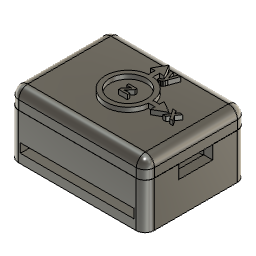
Tremolomter accel case (Autodesk Fusion 360 design; units mm, degrees)
Autodesk Fusion 360 part; units mm, degrees
sketch "Sketch1" plane through (0, 0, 0) normal (0, 0, 1) x (1, 0, 0)
  line L0 (0, 0) -> (29.9, 0)
  line L1 (29.9, 0) -> (29.9, 22.28)
  line L2 (29.9, 22.28) -> (0, 22.28)
  line L3 (0, 22.28) -> (0, 0)
  dimension "d4" = 29.9
  dimension "d5" = 22.28
  constraint horizontal L0
  constraint vertical L1
  constraint horizontal L2
  constraint vertical L3
  constraint coincident L0.start L3.end
  measures "d4" distance of L0.start L0.end
  measures "d5" distance of L0.start L2.end
extrude "Extrude1" add sketch "Sketch1" along normal blind 2 makes body 1
sketch "Sketch2" plane through (0, 0, 2) normal (0, 0, 1) x (-1, 0, 0)
  line L0 (0, -22.28) -> (0, 0)
  line L1 (0, 0) -> (-29.9, 0)
  line L2 (-29.9, 0) -> (-29.9, -22.28)
  line L3 (-29.9, -22.28) -> (0, -22.28)
  line L4 (-2, -2) -> (-27.9, -2)
  line L5 (-27.9, -2) -> (-27.9, -20.28)
  line L6 (-27.9, -20.28) -> (-2, -20.28)
  line L7 (-2, -20.28) -> (-2, -2)
  dimension "d9" = 25.9
  dimension "d10" = 18.28
  dimension "d11" = 2
  dimension "d12" = 2
  constraint horizontal L4
  constraint vertical L5
  constraint horizontal L6
  constraint vertical L7
  measures "d9" distance of L4.start L4.end
  measures "d10" distance of L4.start L6.end
  measures "d11" distance of L0 L7
  measures "d12" distance of L1 L4
extrude "Extrude2" add sketch "Sketch2" along normal blind 5 bodies 1
sketch "Sketch3" plane through (29.9, 0, 0) normal (1, 0, 0) x (0, 1, 0)
  line L0 (0, 0) -> (22.28, 0)
  line L1 (22.28, 0) -> (22.28, 7)
  line L2 (22.28, 7) -> (0, 7)
  line L3 (0, 7) -> (0, 0)
  line L4 (7.39, 4) -> (14.89, 4)
  line L5 (14.89, 4) -> (14.89, 7)
  line L6 (14.89, 7) -> (7.39, 7)
  line L7 (7.39, 7) -> (7.39, 4)
  dimension "d17" = 7.5
  dimension "d18" = 3
  dimension "d19" = 4
  dimension "d20" = 7.39
  constraint horizontal L4
  constraint vertical L5
  constraint horizontal L6
  constraint vertical L7
  measures "d17" distance of L4.start L4.end
  measures "d18" distance of L4.start L6.end
  measures "d19" distance of L0 L4
  measures "d20" distance of L3 L7
extrude "Extrude3" cut sketch "Sketch3" against normal blind 14 contours L2 L4 L5 L6 L7 bodies 1
sketch "Sketch4" plane through (0, 0, 2) normal (0, 0, 1) x (-1, 0, 0)
  line L0 (-2, -2) -> (-27.9, -2)
  line L1 (-27.9, -2) -> (-27.9, -20.28)
  line L2 (-27.9, -20.28) -> (-2, -20.28)
  line L3 (-2, -20.28) -> (-2, -2)
  circle A0 centre (-4.54, -17.74) radius 1
  circle A1 centre (-25.36, -17.74) radius 1
  circle A2 centre (-4.54, -4.54) radius 1
  circle A3 centre (-25.36, -4.54) radius 1
  dimension "d26" = 2
  dimension "d27" = 2.54
  dimension "d28" = 2.54
  dimension "d29" = 2
  dimension "d30" = 2.54
  dimension "d31" = 2.54
  dimension "d32" = 2
  dimension "d33" = 2.54
  dimension "d34" = 2.54
  dimension "d35" = 2
  dimension "d36" = 2.54
  dimension "d37" = 2.54
  measures "d26" diameter of A0
  measures "d27" distance of L2 A0.centre
  measures "d28" distance of L3 A0.centre
  measures "d29" diameter of A1
  measures "d30" distance of L2 A1.centre
  measures "d31" distance of L1 A1.centre
  measures "d32" diameter of A2
  measures "d33" distance of L3 A2.centre
  measures "d34" distance of L0 A2.centre
  measures "d35" diameter of A3
  measures "d36" distance of L0 A3.centre
  measures "d37" distance of L1 A3.centre
extrude "Extrude4" add sketch "Sketch4" along normal blind 3 contours A0 | A1 | A2 | A3 bodies 1
extrude "Extrude5" add 1 faces at (9.9667, 14.8533, 0) along direction (0, 0, -1) blind 3 on bodies 1 bodies 1
sketch "Sketch5" plane through (0, 22.28, 0) normal (0, 1, 0) x (-1, 0, 0)
  line L0 (0, -3) -> (0, 7)
  line L1 (0, 7) -> (-29.9, 7)
  line L2 (-29.9, 7) -> (-29.9, -3)
  line L3 (-29.9, -3) -> (0, -3)
  line L4 (-27.45, -1) -> (-2.45, -1)
  line L5 (-2.45, -1) -> (-2.45, 1)
  line L6 (-2.45, 1) -> (-27.45, 1)
  line L7 (-27.45, 1) -> (-27.45, -1)
  dimension "d46" = 25
  dimension "d47" = 2
  dimension "d48" = 2.45
  dimension "d49" = 2
  constraint horizontal L4
  constraint vertical L5
  constraint horizontal L6
  constraint vertical L7
  measures "d46" distance of L4.start L4.end
  measures "d47" distance of L4.start L6.end
  measures "d48" distance of L2 L7
  measures "d49" distance of L3 L4
extrude "Extrude6" cut sketch "Sketch5" against normal blind 36 contours L4 L5 L6 L7 bodies 1
sketch "Sketch6" plane through (0, 0, 7) normal (0, 0, 1) x (-1, 0, 0)
  line L0 (-2, -2) -> (-2, -20.28)
  line L1 (-2, -20.28) -> (-27.9, -20.28)
  line L2 (-27.9, -7.39) -> (-27.9, -2)
  line L3 (-27.9, -2) -> (-2, -2)
  line L4 (-29.9, -22.28) -> (0, -22.28)
  line L5 (0, -22.28) -> (0, 0)
  line L6 (0, 0) -> (-29.9, 0)
  line L7 (-29.9, -14.89) -> (-29.9, -22.28)
  line L8 (-1, -21.28) -> (-2, -21.28)
  line L9 (-2, -21.28) -> (-2, -1)
  line L10 (-2, -1) -> (-1, -1)
  line L11 (-1, -1) -> (-1, -21.28)
  line L12 (-2, -0.9462) -> (-27.9, -0.9462)
  line L13 (-27.9, -0.9462) -> (-27.9, -2)
  line L14 (-27.9, -2) -> (-2, -2)
  line L15 (-2, -2) -> (-2, -0.9462)
  line L16 (-27.9, -21.28) -> (-28.9, -21.28)
  line L17 (-28.9, -21.28) -> (-28.9, -1)
  line L18 (-28.9, -1) -> (-27.9, -1)
  line L19 (-27.9, -1) -> (-27.9, -21.28)
  line L20 (-2, -20.28) -> (-27.9, -20.28)
  line L21 (-27.9, -20.28) -> (-27.9, -21.28)
  line L22 (-27.9, -21.28) -> (-2, -21.28)
  line L23 (-2, -21.28) -> (-2, -20.28)
  line L24 (-29.9, -7.39) -> (-27.9, -7.39)
  line L25 (-27.9, -20.28) -> (-27.9, -14.89)
  line L26 (-27.9, -14.89) -> (-29.9, -14.89)
  line L27 (-29.9, 0) -> (-29.9, -7.39)
  dimension "d54" = 1
  dimension "d55" = 20.28
  dimension "d56" = 1
  dimension "d57" = 1
  dimension "d58" = 25.9
  dimension "d59" = 2
  dimension "d60" = 1
  dimension "d61" = 20.28
  dimension "d62" = 1
  dimension "d63" = 25.9
  dimension "d64" = 1
  dimension "d65" = 2
  dimension "d66" = 1
  constraint horizontal L8
  constraint vertical L9
  constraint horizontal L10
  constraint vertical L11
  constraint horizontal L12
  constraint vertical L13
  constraint horizontal L14
  constraint vertical L15
  constraint horizontal L16
  constraint vertical L17
  constraint horizontal L18
  constraint vertical L19
  constraint coincident L2 L16.start
  constraint horizontal L20
  constraint vertical L21
  constraint horizontal L22
  constraint vertical L23
  measures "d54" distance of L8.start L8.end
  measures "d55" distance of L8.start L10.end
  measures "d56" distance of L5 L11
  measures "d57" distance of L4 L8
  measures "d58" distance of L12.start L12.end
  measures "d59" distance of L5 L15
  measures "d60" distance of L16.start L16.end
  measures "d61" distance of L16.start L18.end
  measures "d62" distance of L4 L16
  measures "d63" distance of L0.end L1.end
  measures "d64" distance of L0.end L8.end
  measures "d65" distance of L5 L23
  measures "d66" distance of L4 L22
extrude "Extrude7" add sketch "Sketch6" along normal blind 2 contours L0 L8 L9 L10 L11 L15 L23 | L3 L9 L12 L13 L14 L15 L19 | L1 L9 L19 L20 L21 L22 L23 | L2 L13 L17 L18 L19 L24 | L16 L17 L19 L21 L25 L26 | L17 L19 L24 L26 bodies 1
ref_plane "WorkPlane1" through (14.95, 11.1131, 9) normal (0, 0, 1) x (1, 0, 0)
sketch "Sketch7" plane through (14.7, 10.8631, 9) normal (0, 0, 1) x (1, 0, 0)
  line L0 (-14.644, -10.8373) -> (15.256, -10.8373)
  line L1 (15.256, -10.8373) -> (15.256, 11.4427)
  line L2 (15.256, 11.4427) -> (-14.644, 11.4427)
  line L3 (-14.644, 11.4427) -> (-14.644, -10.8373)
  dimension "d70" = 29.9
  dimension "d71" = 22.28
  constraint horizontal L0
  constraint vertical L1
  constraint horizontal L2
  constraint vertical L3
  measures "d70" distance of L0.start L0.end
  measures "d71" distance of L0.start L2.end
extrude "Extrude8" add sketch "Sketch7" along normal blind 2 separate body makes body 2
sketch "Sketch8" plane through (0, 0, 9) normal (0, 0, -1) x (1, 0, 0)
  line L0 (0.056, -0.0258) -> (0.056, -22.3058)
  line L1 (0.056, -22.3058) -> (29.956, -22.3058)
  line L2 (29.956, -22.3058) -> (29.956, -0.0258)
  line L3 (29.956, -0.0258) -> (0.056, -0.0258)
  line L4 (1.056, -1.0258) -> (28.956, -1.0258)
  line L5 (28.956, -1.0258) -> (28.956, -21.3058)
  line L6 (28.956, -21.3058) -> (1.056, -21.3058)
  line L7 (1.056, -21.3058) -> (1.056, -1.0258)
  dimension "d74" = 27.9
  dimension "d75" = 20.28
  dimension "d76" = 1
  dimension "d77" = 1
  constraint horizontal L4
  constraint vertical L5
  constraint horizontal L6
  constraint vertical L7
  measures "d74" distance of L4.start L4.end
  measures "d75" distance of L4.start L6.end
  measures "d76" distance of L0 L7
  measures "d77" distance of L3 L4
extrude "Extrude9" add sketch "Sketch8" along normal blind 2 bodies 2
fillet "Fillet1" radius 2 12 edges at (29.9, 22.28, 2) (0, 22.28, 2) (29.9, 0, 2) (0, 0, 2) (29.956, 22.3058, 9) (15.006, 22.3058, 11) (29.956, 11.1658, 11) (0.056, 11.1658, 11) (15.006, 0.0258, 11) (0.056, 22.3058, 9) (29.956, 0.0258, 9) (0.056, 0.0258, 9) on bodies 1 2
sketch "Sketch9" plane through (0, 0, 11) normal (0, 0, 1) x (-1, 0, 0)
  line L0 (-2.056, -20.3058) -> (-2.056, -2.0258)
  line L1 (-2.056, -2.0258) -> (-27.956, -2.0258)
  line L2 (-27.956, -2.0258) -> (-27.956, -20.3058)
  line L3 (-27.956, -20.3058) -> (-2.056, -20.3058)
  circle A0 centre (-15.006, -11.1658) radius 5
  circle A1 centre (-15.006, -11.1658) radius 4
  line L4 (-19.006, -11.6658) -> (-22.506, -11.6658)
  line L5 (-22.506, -11.6658) -> (-22.506, -10.6658)
  line L6 (-22.506, -10.6658) -> (-19.006, -10.6658)
  line L7 (-19.006, -10.6658) -> (-19.006, -11.6658)
  line L8 (-19.006, -10.6658) -> (-15.006, -10.6658) construction
  line L9 (-14.506, -15.1658) -> (-15.506, -15.1658)
  line L10 (-15.506, -15.1658) -> (-15.506, -18.6658)
  line L11 (-15.506, -18.6658) -> (-14.506, -18.6658)
  line L12 (-14.506, -18.6658) -> (-14.506, -15.1658)
  line L13 (-15.006, -18.6658) -> (-15.006, -20.1658)
  line L14 (-15.006, -20.1658) -> (-13.506, -17.5677)
  line L15 (-15.006, -20.1658) -> (-13.006, -20.1658) construction
  line L16 (-15.006, -20.1658) -> (-16.506, -17.5677)
  line L17 (-15.006, -20.1658) -> (-17.006, -20.1658) construction
  line L18 (-13.506, -17.5677) -> (-16.506, -17.5677)
  line L19 (-22.506, -11.1658) -> (-24.006, -11.1658)
  line L20 (-24.006, -11.1658) -> (-21.4079, -12.6658)
  line L21 (-24.006, -11.1658) -> (-21.006, -11.1658) construction
  line L22 (-24.006, -11.1658) -> (-21.4079, -9.6658)
  line L23 (-24.006, -11.1658) -> (-21.006, -11.1658) construction
  line L24 (-21.4079, -12.6658) -> (-21.4079, -9.6658)
  dimension "d84" = 10
  dimension "d85" = 9.14
  dimension "d86" = 12.95
  dimension "d88" = 8
  dimension "d89" = 12.95
  dimension "d90" = 9.14
  dimension "d93" = 3.5
  dimension "d94" = 1
  dimension "d95" = 5.45
  dimension "d96" = 9.64
  dimension "d101" = 1
  dimension "d102" = 3.5
  dimension "d103" = 12.45
  dimension "d104" = 13.14
  dimension "d110" = 1.5
  dimension "d111" = 60
  dimension "d112" = 3
  dimension "d113" = 60
  dimension "d114" = 3
  dimension "d124" = 1.5
  dimension "d125" = 30
  dimension "d126" = 3
  dimension "d127" = 3
  dimension "d128" = 30
  constraint horizontal L4
  constraint vertical L5
  constraint horizontal L6
  constraint vertical L7
  constraint horizontal L8
  constraint horizontal L9
  constraint vertical L10
  constraint horizontal L11
  constraint vertical L12
  constraint midpoint L11 L13.start
  constraint perpendicular L11 L13
  constraint horizontal L15
  constraint horizontal L17
  constraint midpoint L5 L19.start
  constraint perpendicular L5 L19
  constraint horizontal L21
  constraint horizontal L23
  measures "d84" diameter of A0
  measures "d85" distance of L1 A0.centre
  measures "d86" distance of L2 A0.centre
  measures "d88" diameter of A1
  measures "d89" distance of L2 A0.centre
  measures "d90" distance of L1 A0.centre
  measures "d93" distance of L4.start L4.end
  measures "d94" distance of L4.start L6.end
  measures "d95" distance of L2 L5
  measures "d96" distance of L1 L4
  measures "d101" distance of L9.start L9.end
  measures "d102" distance of L9.start L11.end
  measures "d103" distance of L2 L10
  measures "d104" distance of L1 L9
  measures "d110" distance of L13.start L13.end
  measures "d111" angle of L14 L15
  measures "d112" distance of L13.end L14.end
  measures "d113" angle of L16 L17
  measures "d114" distance of L13.end L16.end
  measures "d124" distance of L19.start L19.end
  measures "d125" angle of L20 L21
  measures "d126" distance of L19.end L20.end
  measures "d127" distance of L19.end L22.end
  measures "d128" angle of L22 L23
sketch "Sketch10" plane through (0, 0, 11) normal (0, 0, 1) x (-1, 0, 0)
  line L0 (-2.056, -20.3058) -> (-2.056, -2.0258)
  line L1 (-2.056, -2.0258) -> (-27.956, -2.0258)
  line L2 (-27.956, -2.0258) -> (-27.956, -20.3058)
  line L3 (-27.956, -20.3058) -> (-2.056, -20.3058)
  line L4 (-23.725, -12.0889) -> (-25.1971, -12.0925) construction
  line L5 (-25.1971, -12.0925) -> (-25.1928, -13.8365) construction
  line L6 (-25.1928, -13.8365) -> (-23.7208, -13.8329) construction
  line L7 (-23.7208, -13.8329) -> (-23.725, -12.0889) construction
  line L8 (-16.2107, -18.9407) -> (-17.9786, -18.9407) construction
  line L9 (-17.9786, -18.9407) -> (-17.9786, -20.8846) construction
  line L10 (-17.9786, -20.8846) -> (-16.2107, -20.8846) construction
  line L11 (-16.2107, -20.8846) -> (-16.2107, -18.9407) construction
  line L12 (-14.0697, -10.17) -> (-16.0697, -10.17) construction
  line L13 (-16.0697, -10.17) -> (-16.0697, -12.17) construction
  line L14 (-16.0697, -12.17) -> (-14.0697, -12.17) construction
  line L15 (-14.0697, -12.17) -> (-14.0697, -10.17) construction
  dimension "d119" = 3
  dimension "d120" = 3
  dimension "d121" = 3
  text T0 "x" font "Arial" height 3 bold align left top in box 1.472 x 1.744 at (-23.725, -12.0889) x (-0.999997, -0.002422) y (0.002422, -0.999997) spacing 1 kerned
  text T1 "y" font "Arial" height 3 bold align left top in box 1.7678 x 1.9439 at (-16.2107, -18.9407) x (-1, 0) y (0, -1) spacing 1 kerned
  text T2 "z" font "Arial" height 3 bold align left top in box 2 x 2 at (-14.0697, -10.17) x (-1, 0) y (0, -1) spacing 1 kerned
extrude "Extrude12" add sketch "Sketch9" sketch "Sketch10" along normal blind 1 contours A0 A1 L6 L7 L9 L12 | A0 L4 L6 L7 | A0 L4 L6 L24 | A0 L10 L12 L18 | A0 L9 L10 L12 | A0 A1 L4 L7 L9 L10 | L4 L5 L6 L24 | L5 L6 L19 L22 L24 | L11 L12 L13 L14 L18 | L10 L11 L12 L18 | L4 L5 L19 L20 L24 | L10 L11 L13 L16 L18 of sketch 2 text T0 T1 T2 bodies 2
equation "Accel_Board_Width = 18.28 mm"
equation "Accel_Board_Length = 25.9 mm"
equation "Accel_Board_Height = 5 mm"
equation "d4 = Accel_Board_Length + 2 * Wall_Thickness"
equation "d5 = Accel_Board_Width + 2 * Wall_Thickness"
equation "Wall_Thickness = 2 mm"
equation "d7 = Wall_Thickness"
equation "d9 = Accel_Board_Length"
equation "d10 = Accel_Board_Width"
equation "d11 = Wall_Thickness"
equation "d12 = Wall_Thickness"
equation "d13 = Accel_Board_Height"
equation "Connector_Width = 7.5 mm"
equation "Connector_Height = 3 mm"
equation "d17 = Connector_Width"
equation "d18 = Connector_Height"
equation "d19 = Wall_Thickness + Accel_Board_Panel_Height"
equation "d20 = ( ( 2 * Wall_Thickness + Accel_Board_Width ) / 2 ) - ( Connector_Width / 2 )"
equation "Accel_Board_Panel_Height = 2 mm"
equation "Screw_Hole_Distance_From_Edge = 2.54 mm"
equation "Screw_Hole_Pin_Radius = 2 mm"
equation "d26 = Screw_Hole_Pin_Radius"
equation "d27 = Screw_Hole_Distance_From_Edge"
equation "d28 = Screw_Hole_Distance_From_Edge"
equation "d29 = Screw_Hole_Pin_Radius"
equation "d30 = Screw_Hole_Distance_From_Edge"
equation "d31 = Screw_Hole_Distance_From_Edge"
equation "d32 = Screw_Hole_Pin_Radius"
equation "d33 = Screw_Hole_Distance_From_Edge"
equation "d34 = Screw_Hole_Distance_From_Edge"
equation "d35 = Screw_Hole_Pin_Radius"
equation "d36 = Screw_Hole_Distance_From_Edge"
equation "d37 = Screw_Hole_Distance_From_Edge"
equation "Screw_Hole_Pin_Hight = 3 mm"
equation "d39 = Screw_Hole_Pin_Hight"
equation "Lock_Height = 3 mm"
equation "Lock_Track_Height = 2 mm"
equation "Lock_Track_Width = 25 mm"
equation "d44 = Lock_Height"
equation "d46 = Lock_Track_Width"
equation "d47 = Lock_Track_Height"
equation "d48 = ( ( 2 * Wall_Thickness + Accel_Board_Length ) / 2 ) - ( Lock_Track_Width / 2 )"
equation "d49 = Wall_Thickness"
equation "Locking_Track_Width = Wall_Thickness / 2"
equation "Locking_Track_Height = 2 mm"
equation "d54 = Locking_Track_Width"
equation "d55 = Accel_Board_Width + 2 * Wall_Thickness - 2 * Locking_Track_Width"
equation "d56 = Locking_Track_Width"
equation "d57 = Locking_Track_Width"
equation "d58 = Accel_Board_Length + 2 * Wall_Thickness - 4 * Locking_Track_Width"
equation "d59 = 2 * Locking_Track_Width"
equation "d60 = Locking_Track_Width"
equation "d61 = Accel_Board_Width + 2 * Wall_Thickness - 2 * Locking_Track_Width"
equation "d62 = Locking_Track_Width"
equation "d63 = Accel_Board_Length"
equation "d64 = Locking_Track_Width"
equation "d65 = 2 * Locking_Track_Width"
equation "d66 = Locking_Track_Width"
equation "d67 = Locking_Track_Height"
equation "d70 = 2 * Wall_Thickness + Accel_Board_Length"
equation "d71 = 2 * Wall_Thickness + Accel_Board_Width"
equation "d72 = Wall_Thickness"
equation "d74 = Accel_Board_Length + 2 * Wall_Thickness - 2 * Locking_Track_Width"
equation "d75 = Accel_Board_Width + 2 * Wall_Thickness - 2 * Locking_Track_Width"
equation "d76 = Locking_Track_Width"
equation "d77 = Locking_Track_Width"
equation "d78 = Locking_Track_Height"
equation "Fillet_Radius = 2 mm"
equation "d82 = Fillet_Radius"
equation "Direction_Sign_Cricle_Radius = 10 mm"
equation "d84 = Direction_Sign_Cricle_Radius"
equation "d85 = Accel_Board_Width / 2"
equation "d86 = Accel_Board_Length / 2"
equation "Direction_Sign_Inner_Cricle_Radius = 8 mm"
equation "d88 = Direction_Sign_Inner_Cricle_Radius"
equation "d89 = Accel_Board_Length / 2"
equation "d90 = Accel_Board_Width / 2"
equation "Direction_Sign_Arrow_Base_Length = 3.5 mm"
equation "Direction_Sign_Arrow_Base_Width = 1 mm"
equation "d93 = Direction_Sign_Arrow_Base_Length"
equation "d94 = Direction_Sign_Arrow_Base_Width"
equation "d95 = ( ( Accel_Board_Length - Direction_Sign_Inner_Cricle_Radius ) / 2 ) - Direction_Sign_Arrow_Base_Length"
equation "d96 = ( Accel_Board_Width + Direction_Sign_Arrow_Base_Width ) / 2"
equation "Direction_Sign_Arrow_Top_Width = 3 mm"
equation "Direction_Sign_Arrow_Top_Length = 1.5 mm"
equation "d101 = Direction_Sign_Arrow_Base_Width"
equation "d102 = Direction_Sign_Arrow_Base_Length"
equation "d103 = ( Accel_Board_Length / 2 ) - ( Direction_Sign_Arrow_Base_Width / 2 )"
equation "d104 = ( Accel_Board_Width + Direction_Sign_Inner_Cricle_Radius ) / 2"
equation "d110 = Direction_Sign_Arrow_Top_Length"
equation "d111 = 90 deg - 30 deg"
equation "d112 = 2 * Direction_Sign_Arrow_Top_Length"
equation "d114 = 2 * Direction_Sign_Arrow_Top_Length"
equation "Direction_Sign_Height = 1 mm"
equation "Letter_Size = 3 mm"
equation "d119 = Letter_Size"
equation "d120 = Letter_Size"
equation "d121 = Letter_Size"
equation "d124 = Direction_Sign_Arrow_Top_Length"
equation "d126 = 2 * Direction_Sign_Arrow_Top_Length"
equation "d127 = 2 * Direction_Sign_Arrow_Top_Length"
equation "d129 = Direction_Sign_Height"
named bodies: "Boks", "Lokk"
